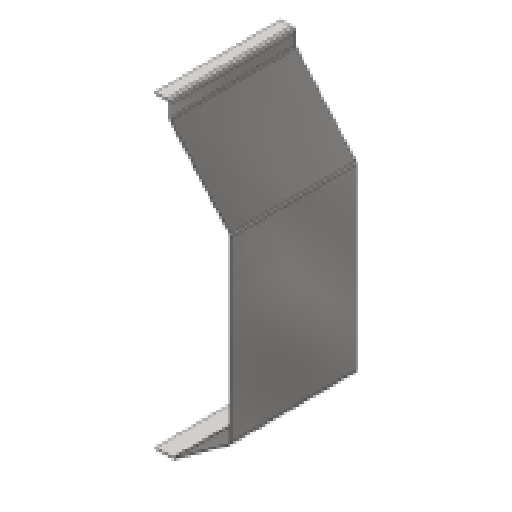
# Autodesk Inventor part: skidPlateV1
Saved by Autodesk Inventor 2025 (Build 290162000, 162)
## iProperties
Created: 2024-12-14
Part Number: skidPlateV1
Material: Stainless Steel
Document SubType Name: Modeling
Designer: derm
Density: 8 g/cm^3
Appearance: Stainless - Brushed
Author: derm
Autodesk Inventor part; units mm, degrees
ref_plane "YZ Plane" through (0, 0, 0) normal (1, 0, 0) x (0, 1, 0)
ref_plane "XZ Plane" through (0, 0, 0) normal (0, 1, 0) x (-1, 0, 0)
ref_plane "XY Plane" through (0, 0, 0) normal (0, 0, 1) x (1, 0, 0)
sketch "Sketch1" plane through (0, 0, 0) normal (0, 0, 1) x (1, 0, 0)
  line L0 (12.58, -266.7) -> (12.58, -12.7) projected
  line L1 (12.6094, 30.4615) -> (-104.0379, 164.6489) projected
  line L2 (-101.051, 167.6239) -> (-101.051, 171.0791) projected
  line L3 (-101.051, 183.7761) -> (-101.051, 187.2313) projected
  line L4 (2.2104, -312.663) -> (11.2162, -295.0088) projected
  line L5 (2.2104, -312.663) -> (-30.82, -336.6137) projected
  line L6 (-87.8643, -376.8499) -> (-98.4679, -380.082) projected
  line L7 (2.14, -312.5659) -> (-85.2529, -375.9353) projected
  line L8 (-103.9473, -380.8694) -> (-107.4025, -380.8694) projected
  line L9 (-120.0995, -380.8694) -> (-123.5547, -380.8694) projected
  line L10 (-120.0995, 190.1276) -> (-123.5547, 190.1276) construction
  line L11 (-101.051, 189.8019) -> (-116.705, 189.8019) construction
  line L12 (-126.451, -355.4694) -> (-126.451, 254.1306) construction
  line L13 (-126.451, 189.8019) -> (-101.051, 189.8019)
  line L14 (12.6094, 30.4615) -> (12.6094, -304.9744)
  line L15 (12.6094, -304.9744) -> (-92.0576, -380.8694)
  line L16 (-92.0576, -380.8694) -> (-126.451, -380.8694)
  line L17 (12.6094, 30.4615) -> (-101.051, 161.2129)
  line L18 (-101.051, 161.2129) -> (-101.051, 189.8019)
  line L19 (-126.451, 191.4275) -> (-99.4254, 191.4275)
  line L20 (-99.4254, 191.4275) -> (-99.4254, 161.8207)
  line L21 (-99.4254, 161.8207) -> (14.235, 31.0693)
  line L22 (14.235, 31.0693) -> (14.235, -305.8037)
  line L23 (14.235, -305.8037) -> (-91.5302, -382.495)
  line L24 (-91.5302, -382.495) -> (-126.451, -382.495)
  line L25 (-126.451, 189.8019) -> (-126.451, 191.4275)
  line L26 (-126.451, -382.495) -> (-126.451, -380.8694)
  point P0 (0, 0)
  dimension "d0" = 1.6256
  constraints: 28 end point, 3 perpendicular, 3 point on line, 2 collinear, 2 vertical, 5 other
  measures "d0" distance between parallel lines of L19 L13
extrude "Extrusion1" add sketch "Sketch1" against normal blind 234
fillet "Fillet1" radius 5 5 edges at (-101.051, 189.8019, -117) (-99.4254, 161.8207, -117) (12.6094, 30.4615, -117) (12.6094, -304.9744, -117) (-92.0576, -380.8694, -117)
fillet "Fillet2" radius 7 5 edges at (-91.5302, -382.495, -117) (14.235, -305.8037, -117) (14.235, 31.0693, -117) (-101.051, 161.2129, -117) (-99.4254, 191.4275, -117)
body "Solid1"
